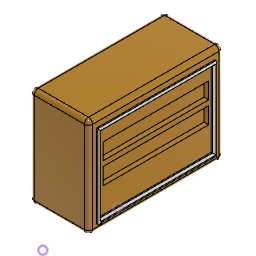
batch-3 19k418 edp (Autodesk Fusion 360 design; units mm, degrees)
Autodesk Fusion 360 part; units mm, degrees
sketch "Sketch1" plane through (0, 0, 0) normal (1, 0, 0) x (0, 1, 0)
  line L0 (-70, 40) -> (160, 40)
  line L1 (160, 40) -> (160, -130)
  line L2 (160, -130) -> (-70, -130)
  line L3 (-70, -130) -> (-70, 40)
  dimension "d1" = 230
  dimension "d2" = 170
  constraint horizontal L0
  constraint vertical L1
  constraint horizontal L2
  constraint vertical L3
  measures "d1" distance of L0.start L0.end
  measures "d2" distance of L0.start L2.end
extrude "Extrude1" add sketch "Sketch1" along normal blind 100 makes body 1
sketch "Sketch2" plane through (0, 0, -130) normal (0, 0, -1) x (1, 0, 0)
  line L0 (0, 70) -> (0, -160)
  line L1 (0, -160) -> (100, -160)
  line L2 (100, -160) -> (100, 70)
  line L3 (100, 70) -> (0, 70)
  line L4 (90, 60) -> (10, 60)
  line L5 (10, 60) -> (10, -70)
  line L6 (10, -70) -> (90, -70)
  line L7 (90, -70) -> (90, 60)
  line L8 (90, -76.1069) -> (10, -76.1069)
  line L9 (10, -76.1069) -> (10, -150)
  line L10 (10, -150) -> (90, -150)
  line L11 (90, -150) -> (90, -76.1069)
  constraint horizontal L4
  constraint vertical L5
  constraint horizontal L6
  constraint vertical L7
  constraint horizontal L8
  constraint vertical L9
  constraint horizontal L10
  constraint vertical L11
extrude "Extrude2" cut sketch "Sketch2" against normal blind 160 contours L4 L5 L6 L7 | L8 L9 L10 L11 bodies 1
sketch "Sketch3" plane through (0, 0, 0) normal (0, 0, 1) x (1, 0, 0)
  line L0 (89, -59) -> (11, -59)
  line L1 (11, -59) -> (11, 69)
  line L2 (11, 69) -> (89, 69)
  line L3 (89, 69) -> (89, -59)
  line L4 (89, 77) -> (11, 77)
  line L5 (11, 77) -> (11, 148.8018)
  line L6 (11, 148.8018) -> (89, 148.8018)
  line L7 (89, 148.8018) -> (89, 77)
  constraint horizontal L0
  constraint vertical L1
  constraint horizontal L2
  constraint vertical L3
  constraint horizontal L4
  constraint vertical L5
  constraint horizontal L6
  constraint vertical L7
extrude "Extrude3" add sketch "Sketch3" against normal blind 158 separate body makes body 2 at (63, 77, -52.6667) makes body 3 at (11, -16.3333, -52.6667)
move_body "Move1" bodies 3 2 to x (1, 0, 0) y (0, 1, 0) z (0, 0, 1) at (0, 0, -200)
sketch "Sketch4" plane through (0, 0, 0) normal (1, 0, 0) x (0, 1, 0)
shell "Shell1" thickness 2 removed faces 1 at (89, 26.3333, -305.3333) on bodies 3
shell "Shell2" thickness 1 removed faces 1 at (89, 124.8679, -305.3333) on bodies 2
sketch "Sketch5" plane through (0, 0, 0) normal (1, 0, 0) x (0, 1, 0)
  line L0 (-25, -365) -> (-25, -375)
  line L1 (-25, -375) -> (15, -375)
  line L2 (15, -375) -> (15, -365)
  constraint vertical L0
  constraint perpendicular L0 L1
  constraint perpendicular L1 L2
sketch "Sketch6" plane through (0, 0, 0) normal (1, 0, 0) x (0, 1, 0)
pipe "Pipe1" add diameter 5 path "Sketch5" along L2 L1 L0 separate body makes body 4
sketch "Sketch7" plane through (0, 0, 0) normal (1, 0, 0) x (0, 1, 0)
  line L0 (90, -365) -> (90, -375)
  line L1 (90, -375) -> (125, -375)
  line L2 (125, -375) -> (125, -365)
  constraint vertical L0
  constraint perpendicular L0 L1
  constraint perpendicular L1 L2
pipe "Pipe2" add diameter 5 path "Sketch7" along L2 L1 L0 separate body makes body 5
move_body "Move2" bodies 4 5 to x (1, 0, 0) y (0, 1, 0) z (0, 0, 1) at (55, 0, 7)
move_body "Move3" bodies 5 to x (1, 0, 0) y (0, 1, 0) z (0, 0, 1) at (0, 5, 0)
sketch "Sketch8" plane through (100, 0, 0) normal (1, 0, 0) x (0, 1, 0)
  line L0 (-70, -130) -> (160, -130)
  line L1 (160, -130) -> (160, 40)
  line L2 (160, 40) -> (-70, 40)
  line L3 (-70, 40) -> (-70, -130)
  line L4 (-44.62, -1.9949) -> (135.38, -1.9949)
  line L5 (135.38, -1.9949) -> (135.38, -30)
  line L6 (135.38, -30) -> (-44.62, -30)
  line L7 (-44.62, -30) -> (-44.62, -1.9949)
  line L8 (-44.62, -38.601) -> (135.38, -38.601)
  line L9 (135.38, -38.601) -> (135.38, -67.0022)
  line L10 (135.38, -67.0022) -> (-44.62, -67.0022)
  line L11 (-44.62, -67.0022) -> (-44.62, -38.601)
  dimension "d19" = 180
  constraint horizontal L4
  constraint vertical L5
  constraint horizontal L6
  constraint vertical L7
  constraint horizontal L8
  constraint vertical L9
  constraint horizontal L10
  constraint vertical L11
  measures "d19" distance of L4.start L4.end
extrude "Extrude4" cut sketch "Sketch8" against normal blind 8 contours L4 L5 L6 L7 | L8 L9 L10 L11 bodies 1
sketch "Sketch9" plane through (11, 0, 0) normal (-1, 0, 0) x (0, -1, 0)
  line L0 (59, -200) -> (-69, -200)
sketch "Sketch10" plane through (0, 0, 0) normal (0, 0, 1) x (1, 0, 0)
fillet "Fillet1" radius 7 12 edges at (0, 160, -45) (0, 45, 40) (50, 160, 40) (0, -70, -45) (50, -70, 40) (100, -70, -45) (100, 45, 40) (100, 160, -45) (50, 160, -130) (100, 45, -130) (0, 45, -130) (50, -70, -130) on bodies 1
sketch "Sketch11" plane through (100, 0, 0) normal (1, 0, 0) x (0, 1, 0)
  line L0 (135.38, -38.601) -> (135.38, -67.0022)
  line L1 (135.38, -67.0022) -> (-44.62, -67.0022)
  line L2 (-44.62, -67.0022) -> (-44.62, -38.601)
  line L3 (-44.62, -38.601) -> (135.38, -38.601)
  line L4 (135.38, -1.9949) -> (135.38, -30)
  line L5 (135.38, -30) -> (-44.62, -30)
  line L6 (-44.62, -30) -> (-44.62, -1.9949)
  line L7 (-44.62, -1.9949) -> (135.38, -1.9949)
  line L8 (153, 33) -> (-63, 33)
  line L9 (-63, 33) -> (-63, -123)
  line L10 (-63, -123) -> (153, -123)
  line L11 (153, -123) -> (153, 33)
  line L12 (-56.3078, 23.8998) -> (146.2384, 23.8998)
  line L13 (146.2384, 23.8998) -> (146.2384, -118.1296)
  line L14 (146.2384, -118.1296) -> (-56.3078, -118.1296)
  line L15 (-56.3078, -118.1296) -> (-56.3078, 23.8998)
  line L16 (-52.6929, 19.4496) -> (140, 19.4496)
  line L17 (140, 19.4496) -> (140, -110)
  line L18 (140, -110) -> (-52.6929, -110)
  line L19 (-52.6929, -110) -> (-52.6929, 19.4496)
  constraint horizontal L12
  constraint vertical L13
  constraint horizontal L14
  constraint vertical L15
  constraint horizontal L16
  constraint vertical L17
  constraint horizontal L18
  constraint vertical L19
extrude "Extrude1'" add sketch "Sketch11" along normal blind 5 separate body contours L12 L13 L14 L15 makes body 6 in component "Component"
fillet "Fillet1'" radius 3 8 edges at (105, -52.6929, -45.2752) (105, -56.3078, -47.1149) (105, 44.9653, -118.1296) (105, 43.6535, -110) (105, 146.2384, -47.1149) (105, 140, -45.2752) (105, 43.6535, 19.4496) (105, 44.9653, 23.8998) on bodies 6 in component "Component"
move_body "Move4" bodies 3 4 2 5 to x (1, 0, 0) y (0, 1, 0) z (0, 0, 1) at (0, 0, 230)
move_body "Move5" bodies 3 4 2 5 to x (1, 0, 0) y (0, 1, 0) z (0, 0, 1) at (0, 0, -275)
move_body "Move6" bodies 3 2 4 5 to x (1, 0, 0) y (0, 1, 0) z (0, 0, 1) at (0, 0, 100)
move_body "Move7" bodies 2 5 3 4 to x (1, 0, 0) y (0, 1, 0) z (0, 0, 1) at (0, 0, 170)
move_body "Move8" bodies 3 4 2 5 to x (1, 0, 0) y (0, 1, 0) z (0, 0, 1) at (0, 0, 5)
component "Component" placed x (1, 0, 0) y (0, 1, 0) z (0, 0, 1) at (0, 0, 0)
